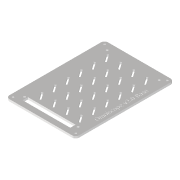
# Autodesk Inventor part: Omniscope_2.0_Base
Saved by Autodesk Inventor 2022 (Build 260153000, 153)
## iProperties
Created: 2022-05-25
Part Number: Omniscope_2.0_Base
Material: Generisch
Document SubType Name: Modeling
Designer: diederichbenedict
Density: 1 g/cm^3
Appearance: Vorgabe
Author: diederichbenedict
Autodesk Inventor part; units mm, degrees
ref_plane "YZ Plane" through (0, 0, 0) normal (1, 0, 0) x (0, 1, 0)
ref_plane "XZ Plane" through (0, 0, 0) normal (0, 1, 0) x (-1, 0, 0)
ref_plane "XY Plane" through (0, 0, 0) normal (0, 0, 1) x (1, 0, 0)
sketch "Skizze1" plane through (0, 0, 0) normal (0, 1, 0) x (-1, 0, 0)
  line L0 (-42.75, -63.75) -> (42.75, -63.75)
  line L1 (42.75, -63.75) -> (42.75, 63.75)
  line L2 (42.75, 63.75) -> (-42.75, 63.75)
  line L3 (-42.75, 63.75) -> (-42.75, -63.75)
  line L4 (-42.75, -63.75) -> (42.75, 63.75) construction
  line L5 (42.75, -63.75) -> (-42.75, 63.75) construction
  line L6 (46.7304, -64.3892) -> (-44.1, -64.3892) projected
  line L7 (46.7304, 68.4528) -> (46.7304, -64.3892) projected
  line L8 (-44.1, 68.4528) -> (46.7304, 68.4528) projected
  line L9 (-44.1, -64.3892) -> (-44.1, 68.4528) projected
  circle A0 centre (-37.9024, -58.852) radius 1.6 projected
  circle A1 centre (-37.75, 58.75) radius 1.6 projected
  circle A2 centre (-30.897, 60.7312) radius 0.5 construction
  circle A3 centre (-28.357, 60.7312) radius 0.5 construction
  circle A4 centre (-25.4992, 60.7312) radius 0.5 construction
  circle A5 centre (-22.9592, 60.7312) radius 0.5 construction
  circle A6 centre (-12.1431, 60.8071) radius 0.5 construction
  circle A7 centre (-9.6031, 60.8071) radius 0.5 construction
  circle A8 centre (-6.7453, 60.8071) radius 0.5 construction
  circle A9 centre (-4.2053, 60.8071) radius 0.5 construction
  circle A10 centre (28.29, -47.2696) radius 1.6 projected
  circle A11 centre (37.5356, -58.7504) radius 1.6 projected
  circle A12 centre (6.8561, 60.8071) radius 0.5 construction
  circle A13 centre (9.3961, 60.8071) radius 0.5 construction
  circle A14 centre (12.2539, 60.8071) radius 0.5 construction
  circle A15 centre (14.7939, 60.8071) radius 0.5 construction
  circle A16 centre (25.7537, 60.8579) radius 0.5 construction
  circle A17 centre (28.2937, 60.8579) radius 0.5 construction
  circle A18 centre (31.1515, 60.8579) radius 0.5 construction
  circle A19 centre (33.6915, 60.8579) radius 0.5 construction
  circle A20 centre (38.9072, 59.8168) radius 1.6 projected
  line L10 (46.7304, -69.3892) -> (-44.1, -69.3892)
  line L11 (-49.1, -64.3892) -> (-49.1, 68.4528)
  line L12 (-44.1, 73.4528) -> (46.7304, 73.4528)
  line L13 (51.7304, 68.4528) -> (51.7304, -64.3892)
  arc A21 (51.7304, 68.4528) -> (46.7304, 73.4528) centre (46.7304, 68.4528) ccw
  arc A22 (-44.1, 73.4528) -> (-49.1, 68.4528) centre (-44.1, 68.4528) ccw
  arc A23 (-49.1, -64.3892) -> (-44.1, -69.3892) centre (-44.1, -64.3892) ccw
  arc A24 (46.7304, -69.3892) -> (51.7304, -64.3892) centre (46.7304, -64.3892) ccw
  line L14 (-33.3052, 57.5577) -> (35.9356, 57.5577)
  line L15 (35.9356, 57.5577) -> (35.9356, 65.2759)
  line L16 (35.9356, 65.2759) -> (-33.3052, 65.2759)
  line L17 (-33.3052, 65.2759) -> (-33.3052, 57.5577)
  line L18 (-33.3052, 57.5577) -> (35.9356, 65.2759) construction
  line L19 (35.9356, 57.5577) -> (-33.3052, 65.2759) construction
  point P0 (0, 0)
  point P1 (1.3152, 61.4168)
  dimension "d0" = 85.5
  dimension "d1" = 127.5
  dimension "d47" = 5
  dimension "d48" = 5
  constraints: 32 end point, 8 point on circle, 8 tangent, 4 centre point, 4 midpoint, 4 parallel, 3 equal radius, 2 horizontal, 2 perpendicular, 3 other
  measures "d0" distance of L2.end L1.end
  measures "d1" distance of L1.end L0.end
  measures "d47" distance between parallel lines of L7 L13
  measures "d48" radius of A21
extrude "Extrusion1" add sketch "Skizze1" along normal blind 3 contours L3 L2 L17 L14 L15 L1 L0 | L6 L9 L8 L7 | A10 | L10 A23 L11 A22 L12 A21 L13 A24
sketch "Skizze8" plane through (0, 3, 0) normal (0, 1, 0) x (1, 0, 0)
  circle A0 centre (-28.29, 47.2696) radius 1.6 projected
  line L0 (-46.7304, -73.4528) -> (44.1, -73.4528) projected
  arc A1 (44.1, -73.4528) -> (49.1, -68.4528) centre (44.1, -68.4528) ccw projected
  line L1 (49.1, -68.4528) -> (49.1, 64.3892) projected
  arc A2 (49.1, 64.3892) -> (44.1, 69.3892) centre (44.1, 64.3892) ccw projected
  line L2 (44.1, 69.3892) -> (-46.7304, 69.3892) projected
  arc A3 (-46.7304, 69.3892) -> (-51.7304, 64.3892) centre (-46.7304, 64.3892) ccw projected
  line L3 (-51.7304, 64.3892) -> (-51.7304, -68.4528) projected
  arc A4 (-51.7304, -68.4528) -> (-46.7304, -73.4528) centre (-46.7304, -68.4528) ccw projected
  line L4 (-32.7356, 53.5165) -> (-24.8933, 42.3165)
  line L5 (-24.8933, 42.3165) -> (-22.8454, 43.7504)
  line L6 (-22.8454, 43.7504) -> (-30.6877, 54.9504)
  line L7 (-30.6877, 54.9504) -> (-32.7356, 53.5165)
  line L8 (-32.7356, 53.5165) -> (-22.8454, 43.7504) construction
  line L9 (-24.8933, 42.3165) -> (-30.6877, 54.9504) construction
  line L10 (-32.7356, 53.5165) -> (-19.0629, 53.5165) construction
  circle A5 centre (-37.5356, 58.7504) radius 1.6 projected
  point P0 (0, 0)
  point P1 (-27.7905, 48.6334)
  dimension "d49" = 55
  dimension "d50" = 2.5
  dimension "d51" = 35
  dimension "d55" = 3.8
  dimension "d57" = 15
  dimension "d58" = 4.8
  constraints: 14 end point, 2 midpoint, 2 parallel, 1 equal length, 1 horizontal, 1 perpendicular
  measures "d49" angle of L4 L10
  measures "d50" distance of L5.end L4.end
  measures "d51" angle of L4 L3
  measures "d55" vertical distance of A5.centre L6.end
  measures "d57" vertical distance of A5.centre L5.end
  measures "d58" horizontal distance of L4.start A5.centre
extrude "Extrusion5" cut sketch "Skizze8" against normal through all contours A0 L4 | A0 L4 L7 L6 L5 picked at (-28.4041, 47.7742)
pattern_linear "Rechteckige Anordnung3" count 6 spacing 19 along (0, 0, 1) count 4 spacing 19 along (1, 0, 0) of "Extrusion5"
sketch "Skizze9" plane through (0, 3, 0) normal (0, 1, 0) x (1, 0, 0)
  line L0 (32.1067, -52.6835) -> (24.2644, -41.4835) projected
  line L1 (24.2644, -41.4835) -> (26.3123, -40.0496) projected
  line L2 (26.3123, -40.0496) -> (34.1546, -51.2496) projected
  line L3 (34.1546, -51.2496) -> (32.1067, -52.6835) projected
  line L4 (32.1067, -33.6835) -> (24.2644, -22.4835) projected
  line L5 (24.2644, -22.4835) -> (26.3123, -21.0496) projected
  line L6 (26.3123, -21.0496) -> (34.1546, -32.2496) projected
  line L7 (34.1546, -32.2496) -> (32.1067, -33.6835) projected
  line L8 (32.1067, -14.6835) -> (24.2644, -3.4835) projected
  line L9 (24.2644, -3.4835) -> (26.3123, -2.0496) projected
  line L10 (26.3123, -2.0496) -> (34.1546, -13.2496) projected
  line L11 (34.1546, -13.2496) -> (32.1067, -14.6835) projected
  line L12 (32.1067, 4.3165) -> (24.2644, 15.5165) projected
  line L13 (24.2644, 15.5165) -> (26.3123, 16.9504) projected
  line L14 (26.3123, 16.9504) -> (34.1546, 5.7504) projected
  line L15 (34.1546, 5.7504) -> (32.1067, 4.3165) projected
  line L16 (32.1067, 23.3165) -> (24.2644, 34.5165) projected
  line L17 (24.2644, 34.5165) -> (26.3123, 35.9504) projected
  line L18 (26.3123, 35.9504) -> (34.1546, 24.7504) projected
  line L19 (34.1546, 24.7504) -> (32.1067, 23.3165) projected
  line L20 (32.1067, 42.3165) -> (24.2644, 53.5165) projected
  line L21 (24.2644, 53.5165) -> (26.3123, 54.9504) projected
  line L22 (26.3123, 54.9504) -> (34.1546, 43.7504) projected
  line L23 (34.1546, 43.7504) -> (32.1067, 42.3165) projected
  line L24 (13.1067, -52.6835) -> (5.2644, -41.4835) projected
  line L25 (5.2644, -41.4835) -> (7.3123, -40.0496) projected
  line L26 (7.3123, -40.0496) -> (15.1546, -51.2496) projected
  line L27 (15.1546, -51.2496) -> (13.1067, -52.6835) projected
  line L28 (13.1067, -33.6835) -> (5.2644, -22.4835) projected
  line L29 (5.2644, -22.4835) -> (7.3123, -21.0496) projected
  line L30 (7.3123, -21.0496) -> (15.1546, -32.2496) projected
  line L31 (15.1546, -32.2496) -> (13.1067, -33.6835) projected
  line L32 (13.1067, -14.6835) -> (5.2644, -3.4835) projected
  line L33 (5.2644, -3.4835) -> (7.3123, -2.0496) projected
  line L34 (7.3123, -2.0496) -> (15.1546, -13.2496) projected
  line L35 (15.1546, -13.2496) -> (13.1067, -14.6835) projected
  line L36 (13.1067, 4.3165) -> (5.2644, 15.5165) projected
  line L37 (5.2644, 15.5165) -> (7.3123, 16.9504) projected
  line L38 (7.3123, 16.9504) -> (15.1546, 5.7504) projected
  line L39 (15.1546, 5.7504) -> (13.1067, 4.3165) projected
  line L40 (13.1067, 23.3165) -> (5.2644, 34.5165) projected
  line L41 (5.2644, 34.5165) -> (7.3123, 35.9504) projected
  line L42 (7.3123, 35.9504) -> (15.1546, 24.7504) projected
  line L43 (15.1546, 24.7504) -> (13.1067, 23.3165) projected
  line L44 (13.1067, 42.3165) -> (5.2644, 53.5165) projected
  line L45 (5.2644, 53.5165) -> (7.3123, 54.9504) projected
  line L46 (7.3123, 54.9504) -> (15.1546, 43.7504) projected
  line L47 (15.1546, 43.7504) -> (13.1067, 42.3165) projected
  line L48 (-5.8933, -52.6835) -> (-13.7356, -41.4835) projected
  line L49 (-13.7356, -41.4835) -> (-11.6877, -40.0496) projected
  line L50 (-11.6877, -40.0496) -> (-3.8454, -51.2496) projected
  line L51 (-3.8454, -51.2496) -> (-5.8933, -52.6835) projected
  line L52 (-5.8933, -33.6835) -> (-13.7356, -22.4835) projected
  line L53 (-13.7356, -22.4835) -> (-11.6877, -21.0496) projected
  line L54 (-11.6877, -21.0496) -> (-3.8454, -32.2496) projected
  line L55 (-3.8454, -32.2496) -> (-5.8933, -33.6835) projected
  line L56 (-5.8933, -14.6835) -> (-13.7356, -3.4835) projected
  line L57 (-13.7356, -3.4835) -> (-11.6877, -2.0496) projected
  line L58 (-11.6877, -2.0496) -> (-3.8454, -13.2496) projected
  line L59 (-3.8454, -13.2496) -> (-5.8933, -14.6835) projected
  line L60 (-5.8933, 4.3165) -> (-13.7356, 15.5165) projected
  line L61 (-13.7356, 15.5165) -> (-11.6877, 16.9504) projected
  line L62 (-11.6877, 16.9504) -> (-3.8454, 5.7504) projected
  line L63 (-3.8454, 5.7504) -> (-5.8933, 4.3165) projected
  line L64 (-5.8933, 23.3165) -> (-13.7356, 34.5165) projected
  line L65 (-13.7356, 34.5165) -> (-11.6877, 35.9504) projected
  line L66 (-11.6877, 35.9504) -> (-3.8454, 24.7504) projected
  line L67 (-3.8454, 24.7504) -> (-5.8933, 23.3165) projected
  line L68 (-5.8933, 42.3165) -> (-13.7356, 53.5165) projected
  line L69 (-13.7356, 53.5165) -> (-11.6877, 54.9504) projected
  line L70 (-11.6877, 54.9504) -> (-3.8454, 43.7504) projected
  line L71 (-3.8454, 43.7504) -> (-5.8933, 42.3165) projected
  line L72 (-24.8933, -52.6835) -> (-32.7356, -41.4835) projected
  line L73 (-32.7356, -41.4835) -> (-30.6877, -40.0496) projected
  line L74 (-30.6877, -40.0496) -> (-22.8454, -51.2496) projected
  line L75 (-22.8454, -51.2496) -> (-24.8933, -52.6835) projected
  line L76 (-24.8933, -33.6835) -> (-32.7356, -22.4835) projected
  line L77 (-32.7356, -22.4835) -> (-30.6877, -21.0496) projected
  line L78 (-30.6877, -21.0496) -> (-22.8454, -32.2496) projected
  line L79 (-22.8454, -32.2496) -> (-24.8933, -33.6835) projected
  line L80 (-24.8933, -14.6835) -> (-32.7356, -3.4835) projected
  line L81 (-32.7356, -3.4835) -> (-30.6877, -2.0496) projected
  line L82 (-30.6877, -2.0496) -> (-22.8454, -13.2496) projected
  line L83 (-22.8454, -13.2496) -> (-24.8933, -14.6835) projected
  line L84 (-24.8933, 4.3165) -> (-32.7356, 15.5165) projected
  line L85 (-32.7356, 15.5165) -> (-30.6877, 16.9504) projected
  line L86 (-30.6877, 16.9504) -> (-22.8454, 5.7504) projected
  line L87 (-22.8454, 5.7504) -> (-24.8933, 4.3165) projected
  line L88 (-24.8933, 23.3165) -> (-32.7356, 34.5165) projected
  line L89 (-32.7356, 34.5165) -> (-30.6877, 35.9504) projected
  line L90 (-30.6877, 35.9504) -> (-22.8454, 24.7504) projected
  line L91 (-22.8454, 24.7504) -> (-24.8933, 23.3165) projected
  line L92 (-30.6877, 54.9504) -> (-22.8454, 43.7504) projected
  line L93 (-22.8454, 43.7504) -> (-24.8933, 42.3165) projected
  line L94 (-24.8933, 42.3165) -> (-32.7356, 53.5165) projected
  line L95 (-32.7356, 53.5165) -> (-30.6877, 54.9504) projected
  line L96 (-46.7304, -73.4528) -> (44.1, -73.4528) projected
  arc A0 (44.1, -73.4528) -> (49.1, -68.4528) centre (44.1, -68.4528) ccw projected
  line L97 (49.1, -68.4528) -> (49.1, 64.3892) projected
  arc A1 (49.1, 64.3892) -> (44.1, 69.3892) centre (44.1, 64.3892) ccw projected
  line L98 (44.1, 69.3892) -> (-46.7304, 69.3892) projected
  arc A2 (-46.7304, 69.3892) -> (-51.7304, 64.3892) centre (-46.7304, 64.3892) ccw projected
  line L99 (-51.7304, 64.3892) -> (-51.7304, -68.4528) projected
  arc A3 (-51.7304, -68.4528) -> (-46.7304, -73.4528) centre (-46.7304, -68.4528) ccw projected
  circle A4 centre (-38.9072, -59.8168) radius 1.6 projected
  circle A5 centre (-37.5356, 58.7504) radius 1.6 projected
  circle A6 centre (37.75, -58.75) radius 1.6 projected
  circle A7 centre (37.9024, 58.852) radius 1.6 projected
  line L100 (33.3052, -57.5577) -> (33.3052, -65.2759) projected
  line L101 (33.3052, -65.2759) -> (-35.9356, -65.2759) projected
  line L102 (-35.9356, -65.2759) -> (-35.9356, -57.5577) projected
  line L103 (-35.9356, -57.5577) -> (33.3052, -57.5577) projected
  point P0 (0, 0)
hole "Bohrung3" at (44.1, 3, 68.4528) at (44.1, 3, -64.3892) at (-46.7304, 3, -64.3892) at (-46.7304, 3, 68.4528) direction (0, -1, 0) diameter 2.8 depth 14 tip angle 118
sketch "Skizze10" plane through (0, 3, 0) normal (0, 1, 0) x (1, 0, 0)
  line L0 (38.6334, -37.4624) -> (38.6334, 40.4783) construction
  line L1 (38.6334, 40.4783) -> (46.1532, 40.4783) construction
  line L2 (46.1532, 40.4783) -> (46.1532, -37.4624) construction
  line L3 (46.1532, -37.4624) -> (38.6334, -37.4624) construction
  spline S0 degree 2 poles (39.4178, -32.7749) (39.8029, -32.4461) (40.9302, -32.0798) (41.6535, -32.0798) knots 0 0 0 1 2 2 2
  spline S1 degree 2 poles (41.6535, -32.0798) (42.3581, -32.0798) (43.4994, -32.4367) (43.8846, -32.7749) knots 0 0 0 1 2 2 2
  spline S2 degree 2 poles (43.8846, -32.7749) (44.2885, -33.1319) (44.6736, -34.0759) (44.6736, -34.6443) knots 0 0 0 1 2 2 2
  spline S3 degree 2 poles (44.6736, -34.6443) (44.6736, -35.2314) (44.2744, -36.1708) (43.8846, -36.5136) knots 0 0 0 1 2 2 2
  spline S4 degree 2 poles (43.8846, -36.5136) (43.4994, -36.8471) (42.3674, -37.2041) (41.6535, -37.2041) knots 0 0 0 1 2 2 2
  spline S5 degree 2 poles (41.6535, -37.2041) (40.9255, -37.2041) (39.817, -36.8424) (39.4178, -36.5089) knots 0 0 0 1 2 2 2
  spline S6 degree 2 poles (39.4178, -36.5089) (39.0326, -36.1708) (38.6334, -35.2267) (38.6334, -34.6443) knots 0 0 0 1 2 2 2
  spline S7 degree 2 poles (38.6334, -34.6443) (38.6334, -34.0525) (39.0467, -33.1037) (39.4178, -32.7749) knots 0 0 0 1 2 2 2
  spline S8 degree 2 poles (41.6535, -32.8829) (41.0805, -32.8829) (40.1928, -33.1319) (39.9016, -33.3573) knots 0 0 0 1 2 2 2
  spline S9 degree 2 poles (39.9016, -33.3573) (39.601, -33.5875) (39.3004, -34.2356) (39.3004, -34.6396) knots 0 0 0 1 2 2 2
  spline S10 degree 2 poles (39.3004, -34.6396) (39.3004, -35.0576) (39.5916, -35.687) (39.9016, -35.9265) knots 0 0 0 1 2 2 2
  spline S11 degree 2 poles (39.9016, -35.9265) (40.1975, -36.1567) (41.0899, -36.4009) (41.6535, -36.4009) knots 0 0 0 1 2 2 2
  spline S12 degree 2 poles (41.6535, -36.4009) (42.7949, -36.4009) (44.0067, -35.4427) (44.0067, -34.6396) knots 0 0 0 1 2 2 2
  spline S13 degree 2 poles (44.0067, -34.6396) (44.0067, -33.8364) (42.7949, -32.8829) (41.6535, -32.8829) knots 0 0 0 1 2 2 2
  line L4 (44.5515, -26.3589) -> (42.034, -26.3589)
  spline S14 degree 2 poles (42.034, -26.3589) (41.7334, -26.3589) (41.2214, -26.4059) (41.0805, -26.481) knots 0 0 0 1 2 2 2
  spline S15 degree 2 poles (41.0805, -26.481) (40.9255, -26.5562) (40.7752, -26.8427) (40.7752, -27.0916) knots 0 0 0 1 2 2 2
  spline S16 degree 2 poles (40.7752, -27.0916) (40.7752, -27.3171) (41.0523, -27.8337) (41.3153, -28.1062) knots 0 0 0 1 2 2 2
  spline S17 degree 2 poles (41.3153, -28.1062) (41.3811, -28.1015) (41.5643, -28.0921) (41.6864, -28.0921) knots 0 0 0 1 2 2 2
  line L5 (41.6864, -28.0921) -> (44.5515, -28.0921)
  line L6 (44.5515, -28.0921) -> (44.5515, -28.8248)
  line L7 (44.5515, -28.8248) -> (42.034, -28.8248)
  spline S18 degree 2 poles (42.034, -28.8248) (41.7334, -28.8248) (41.2214, -28.8718) (41.0805, -28.9469) knots 0 0 0 1 2 2 2
  spline S19 degree 2 poles (41.0805, -28.9469) (40.9255, -29.0221) (40.7752, -29.3086) (40.7752, -29.5575) knots 0 0 0 1 2 2 2
  spline S20 degree 2 poles (40.7752, -29.5575) (40.7752, -29.7924) (41.0711, -30.3137) (41.3012, -30.558) knots 0 0 0 1 2 2 2
  line L8 (41.3012, -30.558) -> (44.5515, -30.558)
  line L9 (44.5515, -30.558) -> (44.5515, -31.2907)
  line L10 (44.5515, -31.2907) -> (40.2022, -31.2907)
  line L11 (40.2022, -31.2907) -> (40.2022, -30.558)
  line L12 (40.2022, -30.558) -> (40.6813, -30.558)
  spline S21 degree 2 poles (40.6813, -30.558) (40.3947, -30.2714) (40.08, -29.7078) (40.08, -29.3696) knots 0 0 0 1 2 2 2
  spline S22 degree 2 poles (40.08, -29.3696) (40.08, -28.9845) (40.4323, -28.388) (40.8316, -28.233) knots 0 0 0 1 2 2 2
  spline S23 degree 2 poles (40.8316, -28.233) (40.4605, -27.8995) (40.08, -27.2701) (40.08, -26.9037) knots 0 0 0 1 2 2 2
  spline S24 degree 2 poles (40.08, -26.9037) (40.08, -26.6219) (40.2538, -26.1616) (40.4511, -25.9925) knots 0 0 0 1 2 2 2
  spline S25 degree 2 poles (40.4511, -25.9925) (40.6484, -25.8188) (41.2402, -25.6262) (41.6864, -25.6262) knots 0 0 0 1 2 2 2
  line L13 (41.6864, -25.6262) -> (44.5515, -25.6262)
  line L14 (44.5515, -25.6262) -> (44.5515, -26.3589)
  line L15 (44.5515, -21.1829) -> (44.5515, -21.9156)
  line L16 (44.5515, -21.9156) -> (42.0715, -21.9156)
  spline S26 degree 2 poles (42.0715, -21.9156) (41.7709, -21.9156) (41.2543, -21.972) (41.0993, -22.0565) knots 0 0 0 1 2 2 2
  spline S27 degree 2 poles (41.0993, -22.0565) (40.9349, -22.1458) (40.7752, -22.4652) (40.7752, -22.7376) knots 0 0 0 1 2 2 2
  spline S28 degree 2 poles (40.7752, -22.7376) (40.7752, -23.01) (41.0664, -23.5877) (41.3012, -23.8648) knots 0 0 0 1 2 2 2
  line L17 (41.3012, -23.8648) -> (44.5515, -23.8648)
  line L18 (44.5515, -23.8648) -> (44.5515, -24.5976)
  line L19 (44.5515, -24.5976) -> (40.2022, -24.5976)
  line L20 (40.2022, -24.5976) -> (40.2022, -23.8648)
  line L21 (40.2022, -23.8648) -> (40.686, -23.8648)
  spline S29 degree 2 poles (40.686, -23.8648) (40.39, -23.5361) (40.08, -22.902) (40.08, -22.545) knots 0 0 0 1 2 2 2
  spline S30 degree 2 poles (40.08, -22.545) (40.08, -21.9062) (40.9255, -21.1829) (41.7287, -21.1829) knots 0 0 0 1 2 2 2
  line L22 (41.7287, -21.1829) -> (44.5515, -21.1829)
  line L23 (44.5515, -19.4075) -> (44.5515, -20.1402)
  line L24 (44.5515, -20.1402) -> (40.2022, -20.1402)
  line L25 (40.2022, -20.1402) -> (40.2022, -19.4075)
  line L26 (40.2022, -19.4075) -> (44.5515, -19.4075)
  line L27 (39.4788, -19.3558) -> (39.4788, -20.1872)
  line L28 (39.4788, -20.1872) -> (38.7179, -20.1872)
  line L29 (38.7179, -20.1872) -> (38.7179, -19.3558)
  line L30 (38.7179, -19.3558) -> (39.4788, -19.3558)
  spline S31 degree 2 poles (44.6548, -17.1576) (44.6548, -17.5945) (44.42, -18.3507) (44.2885, -18.5996) knots 0 0 0 1 2 2 2
  line L31 (44.2885, -18.5996) -> (43.4665, -18.5996)
  line L32 (43.4665, -18.5996) -> (43.4665, -18.562)
  spline S32 degree 2 poles (43.4665, -18.562) (43.5417, -18.4681) (43.7202, -18.2144) (43.8188, -18.0031) knots 0 0 0 1 2 2 2
  spline S33 degree 2 poles (43.8188, -18.0031) (43.908, -17.8199) (44.0396, -17.369) (44.0396, -17.1295) knots 0 0 0 1 2 2 2
  spline S34 degree 2 poles (44.0396, -17.1295) (44.0396, -16.9557) (43.9597, -16.5564) (43.8939, -16.4625) knots 0 0 0 1 2 2 2
  spline S35 degree 2 poles (43.8939, -16.4625) (43.8047, -16.3263) (43.6027, -16.2042) (43.3961, -16.2042) knots 0 0 0 1 2 2 2
  spline S36 degree 2 poles (43.3961, -16.2042) (43.1377, -16.2042) (42.87, -16.486) (42.7808, -16.8476) knots 0 0 0 1 2 2 2
  spline S37 degree 2 poles (42.7808, -16.8476) (42.7479, -16.9885) (42.654, -17.4395) (42.6023, -17.632) knots 0 0 0 1 2 2 2
  spline S38 degree 2 poles (42.6023, -17.632) (42.4567, -18.1299) (41.8555, -18.5808) (41.4281, -18.5808) knots 0 0 0 1 2 2 2
  spline S39 degree 2 poles (41.4281, -18.5808) (40.8363, -18.5808) (40.0988, -17.6931) (40.0988, -16.9604) knots 0 0 0 1 2 2 2
  spline S40 degree 2 poles (40.0988, -16.9604) (40.0988, -16.5987) (40.2773, -15.866) (40.4135, -15.617) knots 0 0 0 1 2 2 2
  line L33 (40.4135, -15.617) -> (41.1979, -15.617)
  line L34 (41.1979, -15.617) -> (41.1979, -15.6546)
  spline S41 degree 2 poles (41.1979, -15.6546) (40.9725, -15.9364) (40.7141, -16.6222) (40.7141, -16.9745) knots 0 0 0 1 2 2 2
  spline S42 degree 2 poles (40.7141, -16.9745) (40.7141, -17.3361) (41.0194, -17.834) (41.3247, -17.834) knots 0 0 0 1 2 2 2
  spline S43 degree 2 poles (41.3247, -17.834) (41.6019, -17.834) (41.8696, -17.5381) (41.9541, -17.2093) knots 0 0 0 1 2 2 2
  spline S44 degree 2 poles (41.9541, -17.2093) (41.9964, -17.0496) (42.0809, -16.6457) (42.1326, -16.4249) knots 0 0 0 1 2 2 2
  spline S45 degree 2 poles (42.1326, -16.4249) (42.2547, -15.9458) (42.8137, -15.4574) (43.2974, -15.4574) knots 0 0 0 1 2 2 2
  spline S46 degree 2 poles (43.2974, -15.4574) (43.5793, -15.4574) (44.0771, -15.6781) (44.2603, -15.8942) knots 0 0 0 1 2 2 2
  spline S47 degree 2 poles (44.2603, -15.8942) (44.4529, -16.1243) (44.6548, -16.7114) (44.6548, -17.1576) knots 0 0 0 1 2 2 2
  spline S48 degree 2 poles (44.6502, -13.0478) (44.6502, -13.4987) (44.373, -14.2455) (44.0912, -14.5133) knots 0 0 0 1 2 2 2
  spline S49 degree 2 poles (44.0912, -14.5133) (43.8141, -14.781) (42.9593, -15.0769) (42.3862, -15.0769) knots 0 0 0 1 2 2 2
  spline S50 degree 2 poles (42.3862, -15.0769) (41.8132, -15.0769) (40.9772, -14.7716) (40.6953, -14.5133) knots 0 0 0 1 2 2 2
  spline S51 degree 2 poles (40.6953, -14.5133) (40.4088, -14.2549) (40.1035, -13.4893) (40.1035, -13.0478) knots 0 0 0 1 2 2 2
  spline S52 degree 2 poles (40.1035, -13.0478) (40.1035, -12.6909) (40.3055, -12.0239) (40.437, -11.7656) knots 0 0 0 1 2 2 2
  line L35 (40.437, -11.7656) -> (41.259, -11.7656)
  line L36 (41.259, -11.7656) -> (41.259, -11.8078)
  spline S53 degree 2 poles (41.259, -11.8078) (41.1932, -11.8877) (41.0241, -12.1319) (40.9349, -12.3057) knots 0 0 0 1 2 2 2
  spline S54 degree 2 poles (40.9349, -12.3057) (40.8597, -12.4607) (40.7423, -12.874) (40.7423, -13.0619) knots 0 0 0 1 2 2 2
  spline S55 degree 2 poles (40.7423, -13.0619) (40.7423, -13.6302) (41.6019, -14.3207) (42.3862, -14.3207) knots 0 0 0 1 2 2 2
  spline S56 degree 2 poles (42.3862, -14.3207) (43.1518, -14.3207) (44.0114, -13.6537) (44.0114, -13.0619) knots 0 0 0 1 2 2 2
  spline S57 degree 2 poles (44.0114, -13.0619) (44.0114, -12.705) (43.7155, -12.0568) (43.4853, -11.8078) knots 0 0 0 1 2 2 2
  line L37 (43.4853, -11.8078) -> (43.4853, -11.7656)
  line L38 (43.4853, -11.7656) -> (44.3073, -11.7656)
  spline S58 degree 2 poles (44.3073, -11.7656) (44.3589, -11.8736) (44.5045, -12.2024) (44.5374, -12.3339) knots 0 0 0 1 2 2 2
  spline S59 degree 2 poles (44.5374, -12.3339) (44.5938, -12.5218) (44.6502, -12.8177) (44.6502, -13.0478) knots 0 0 0 1 2 2 2
  spline S60 degree 2 poles (42.3768, -7.5243) (43.4759, -7.5243) (44.6736, -8.5811) (44.6736, -9.4641) knots 0 0 0 1 2 2 2
  spline S61 degree 2 poles (44.6736, -9.4641) (44.6736, -10.3706) (43.4383, -11.4086) (42.3768, -11.4086) knots 0 0 0 1 2 2 2
  spline S62 degree 2 poles (42.3768, -11.4086) (41.2872, -11.4086) (40.08, -10.3377) (40.08, -9.4641) knots 0 0 0 1 2 2 2
  spline S63 degree 2 poles (40.08, -9.4641) (40.08, -8.5811) (41.2825, -7.5243) (42.3768, -7.5243) knots 0 0 0 1 2 2 2
  spline S64 degree 2 poles (42.3768, -8.2805) (41.5314, -8.2805) (40.7094, -8.8958) (40.7094, -9.4641) knots 0 0 0 1 2 2 2
  spline S65 degree 2 poles (40.7094, -9.4641) (40.7094, -10.0324) (41.5314, -10.6524) (42.3768, -10.6524) knots 0 0 0 1 2 2 2
  spline S66 degree 2 poles (42.3768, -10.6524) (43.1988, -10.6524) (44.0442, -10.0324) (44.0442, -9.4641) knots 0 0 0 1 2 2 2
  spline S67 degree 2 poles (44.0442, -9.4641) (44.0442, -8.9005) (43.2129, -8.2805) (42.3768, -8.2805) knots 0 0 0 1 2 2 2
  spline S68 degree 2 poles (42.2594, -3.1279) (43.3491, -3.1279) (44.6361, -4.166) (44.6361, -4.9597) knots 0 0 0 1 2 2 2
  spline S69 degree 2 poles (44.6361, -4.9597) (44.6361, -5.2838) (44.4858, -5.7817) (44.3308, -6.04) knots 0 0 0 1 2 2 2
  line L39 (44.3308, -6.04) -> (46.1532, -6.04)
  line L40 (46.1532, -6.04) -> (46.1532, -6.7727)
  line L41 (46.1532, -6.7727) -> (40.2022, -6.7727)
  line L42 (40.2022, -6.7727) -> (40.2022, -6.04)
  line L43 (40.2022, -6.04) -> (40.6578, -6.04)
  spline S70 degree 2 poles (40.6578, -6.04) (40.4088, -5.7676) (40.08, -5.1006) (40.08, -4.7108) knots 0 0 0 1 2 2 2
  spline S71 degree 2 poles (40.08, -4.7108) (40.08, -3.964) (41.2637, -3.1279) (42.2594, -3.1279) knots 0 0 0 1 2 2 2
  spline S72 degree 2 poles (42.344, -3.8841) (41.5972, -3.8841) (40.7752, -4.3585) (40.7752, -4.8893) knots 0 0 0 1 2 2 2
  spline S73 degree 2 poles (40.7752, -4.8893) (40.7752, -5.1993) (41.0523, -5.7817) (41.2684, -6.04) knots 0 0 0 1 2 2 2
  line L44 (41.2684, -6.04) -> (43.7389, -6.04)
  spline S74 degree 2 poles (43.7389, -6.04) (43.8752, -5.7535) (43.9785, -5.3449) (43.9785, -5.0819) knots 0 0 0 1 2 2 2
  spline S75 degree 2 poles (43.9785, -5.0819) (43.9785, -4.5135) (43.1424, -3.8841) (42.344, -3.8841) knots 0 0 0 1 2 2 2
  spline S76 degree 2 poles (44.6502, -0.4789) (44.6502, -1.5216) (43.4806, -2.6676) (42.4003, -2.6676) knots 0 0 0 1 2 2 2
  spline S77 degree 2 poles (42.4003, -2.6676) (41.3388, -2.6676) (40.08, -1.5545) (40.08, -0.6574) knots 0 0 0 1 2 2 2
  spline S78 degree 2 poles (40.08, -0.6574) (40.08, -0.2534) (40.3149, 0.3713) (40.5638, 0.6014) knots 0 0 0 1 2 2 2
  spline S79 degree 2 poles (40.5638, 0.6014) (40.8128, 0.8363) (41.5314, 1.0852) (42.0528, 1.0852) knots 0 0 0 1 2 2 2
  line L45 (42.0528, 1.0852) -> (42.452, 1.0852)
  line L46 (42.452, 1.0852) -> (42.452, -1.9255)
  spline S80 degree 2 poles (42.452, -1.9255) (43.2082, -1.9255) (44.0114, -1.1646) (44.0114, -0.4883) knots 0 0 0 1 2 2 2
  spline S81 degree 2 poles (44.0114, -0.4883) (44.0114, -0.2487) (43.9033, 0.2163) (43.8188, 0.4041) knots 0 0 0 1 2 2 2
  spline S82 degree 2 poles (43.8188, 0.4041) (43.7249, 0.6014) (43.5605, 0.8738) (43.4853, 0.9631) knots 0 0 0 1 2 2 2
  line L47 (43.4853, 0.9631) -> (43.4853, 1.0054)
  line L48 (43.4853, 1.0054) -> (44.2838, 1.0054)
  spline S83 degree 2 poles (44.2838, 1.0054) (44.3355, 0.8785) (44.4858, 0.4934) (44.528, 0.3431) knots 0 0 0 1 2 2 2
  spline S84 degree 2 poles (44.528, 0.3431) (44.5891, 0.1317) (44.6502, -0.2158) (44.6502, -0.4789) knots 0 0 0 1 2 2 2
  spline S85 degree 2 poles (41.8931, 0.3713) (41.5972, 0.3619) (41.165, 0.2398) (41.0194, 0.1223) knots 0 0 0 1 2 2 2
  spline S86 degree 2 poles (41.0194, 0.1223) (40.855, -0.0045) (40.6813, -0.4037) (40.6813, -0.6996) knots 0 0 0 1 2 2 2
  spline S87 degree 2 poles (40.6813, -0.6996) (40.6813, -0.9908) (40.855, -1.3995) (41.0241, -1.5686) knots 0 0 0 1 2 2 2
  spline S88 degree 2 poles (41.0241, -1.5686) (41.1979, -1.7329) (41.6159, -1.902) (41.8931, -1.9255) knots 0 0 0 1 2 2 2
  line L49 (41.8931, -1.9255) -> (41.8931, 0.3713)
  line L50 (40.2022, 7.7313) -> (44.5515, 6.0921)
  line L51 (44.5515, 6.0921) -> (44.5515, 5.4346)
  line L52 (44.5515, 5.4346) -> (40.2022, 3.8094)
  line L53 (40.2022, 3.8094) -> (40.2022, 4.6032)
  line L54 (40.2022, 4.6032) -> (43.5511, 5.7915)
  line L55 (43.5511, 5.7915) -> (40.2022, 6.9704)
  line L56 (40.2022, 6.9704) -> (40.2022, 7.7313)
  line L57 (44.5515, 11.7519) -> (44.5515, 8.1776)
  line L58 (44.5515, 8.1776) -> (43.7296, 8.1776)
  spline S89 degree 2 poles (43.7296, 8.1776) (43.3679, 8.5627) (42.6962, 9.2484) (42.3346, 9.5772) knots 0 0 0 1 2 2 2
  spline S90 degree 2 poles (42.3346, 9.5772) (41.6065, 10.2395) (40.7329, 10.7233) (40.2679, 10.7233) knots 0 0 0 1 2 2 2
  spline S91 degree 2 poles (40.2679, 10.7233) (40.0237, 10.7233) (39.6573, 10.573) (39.5399, 10.4368) knots 0 0 0 1 2 2 2
  spline S92 degree 2 poles (39.5399, 10.4368) (39.4225, 10.3006) (39.3051, 9.9436) (39.3051, 9.7275) knots 0 0 0 1 2 2 2
  spline S93 degree 2 poles (39.3051, 9.7275) (39.3051, 9.5209) (39.4084, 9.0981) (39.4882, 8.9056) knots 0 0 0 1 2 2 2
  spline S94 degree 2 poles (39.4882, 8.9056) (39.554, 8.7412) (39.7419, 8.4359) (39.8076, 8.3419) knots 0 0 0 1 2 2 2
  line L59 (39.8076, 8.3419) -> (39.8076, 8.2997)
  line L60 (39.8076, 8.2997) -> (38.981, 8.2997)
  spline S95 degree 2 poles (38.981, 8.2997) (38.8635, 8.5392) (38.6334, 9.3988) (38.6334, 9.7839) knots 0 0 0 1 2 2 2
  spline S96 degree 2 poles (38.6334, 9.7839) (38.6334, 10.5965) (39.4929, 11.5124) (40.2257, 11.5124) knots 0 0 0 1 2 2 2
  spline S97 degree 2 poles (40.2257, 11.5124) (40.5685, 11.5124) (41.1416, 11.3527) (41.3858, 11.2118) knots 0 0 0 1 2 2 2
  spline S98 degree 2 poles (41.3858, 11.2118) (41.6394, 11.0709) (42.1373, 10.6622) (42.3768, 10.4368) knots 0 0 0 1 2 2 2
  spline S99 degree 2 poles (42.3768, 10.4368) (42.7761, 10.0704) (43.6309, 9.1733) (43.8799, 8.9056) knots 0 0 0 1 2 2 2
  line L61 (43.8799, 8.9056) -> (43.8799, 11.7519)
  line L62 (43.8799, 11.7519) -> (44.5515, 11.7519)
  line L63 (44.5515, 13.7716) -> (44.5515, 12.8416)
  line L64 (44.5515, 12.8416) -> (43.443, 12.8416)
  line L65 (43.443, 12.8416) -> (43.443, 13.7716)
  line L66 (43.443, 13.7716) -> (44.5515, 13.7716)
  spline S100 degree 2 poles (41.6535, 18.5484) (43.2129, 18.5484) (44.6736, 17.6418) (44.6736, 16.6978) knots 0 0 0 1 2 2 2
  spline S101 degree 2 poles (44.6736, 16.6978) (44.6736, 15.7396) (43.1847, 14.8425) (41.6582, 14.8425) knots 0 0 0 1 2 2 2
  spline S102 degree 2 poles (41.6582, 14.8425) (40.0894, 14.8425) (38.6381, 15.749) (38.6381, 16.6978) knots 0 0 0 1 2 2 2
  spline S103 degree 2 poles (38.6381, 16.6978) (38.6381, 17.6512) (40.1411, 18.5484) (41.6535, 18.5484) knots 0 0 0 1 2 2 2
  spline S104 degree 2 poles (43.4196, 17.5526) (43.133, 17.6653) (42.25, 17.7593) (41.6535, 17.7593) knots 0 0 0 1 2 2 2
  spline S105 degree 2 poles (41.6535, 17.7593) (41.057, 17.7593) (40.1787, 17.6653) (39.8828, 17.5479) knots 0 0 0 1 2 2 2
  spline S106 degree 2 poles (39.8828, 17.5479) (39.5869, 17.4305) (39.2816, 17.0219) (39.2816, 16.6978) knots 0 0 0 1 2 2 2
  spline S107 degree 2 poles (39.2816, 16.6978) (39.2816, 16.3737) (39.5869, 15.9557) (39.8922, 15.8335) knots 0 0 0 1 2 2 2
  spline S108 degree 2 poles (39.8922, 15.8335) (40.1881, 15.7161) (41.0899, 15.6316) (41.6582, 15.6316) knots 0 0 0 1 2 2 2
  spline S109 degree 2 poles (41.6582, 15.6316) (42.2688, 15.6316) (43.0861, 15.7067) (43.4055, 15.8288) knots 0 0 0 1 2 2 2
  spline S110 degree 2 poles (43.4055, 15.8288) (43.7061, 15.9416) (44.0302, 16.3596) (44.0302, 16.6978) knots 0 0 0 1 2 2 2
  spline S111 degree 2 poles (44.0302, 16.6978) (44.0302, 17.0172) (43.7249, 17.4352) (43.4196, 17.5526) knots 0 0 0 1 2 2 2
  spline S112 degree 2 poles (42.7714, 25.8755) (43.2035, 25.8755) (43.8658, 25.5468) (44.0818, 25.2743) knots 0 0 0 1 2 2 2
  spline S113 degree 2 poles (44.0818, 25.2743) (44.3355, 24.9456) (44.5515, 24.1987) (44.5515, 23.6069) knots 0 0 0 1 2 2 2
  line L67 (44.5515, 23.6069) -> (44.5515, 21.9442)
  line L68 (44.5515, 21.9442) -> (38.7555, 21.9442)
  line L69 (38.7555, 21.9442) -> (38.7555, 23.4801)
  spline S114 degree 2 poles (38.7555, 23.4801) (38.7555, 24.1001) (38.8354, 24.7201) (38.9904, 25.0019) knots 0 0 0 1 2 2 2
  spline S115 degree 2 poles (38.9904, 25.0019) (39.1548, 25.3166) (39.6949, 25.6031) (40.0613, 25.6031) knots 0 0 0 1 2 2 2
  spline S116 degree 2 poles (40.0613, 25.6031) (40.4699, 25.6031) (41.1181, 25.171) (41.3012, 24.7906) knots 0 0 0 1 2 2 2
  line L70 (41.3012, 24.7906) -> (41.3294, 24.7906)
  spline S117 degree 2 poles (41.3294, 24.7906) (41.4703, 25.3072) (42.2171, 25.8755) (42.7714, 25.8755) knots 0 0 0 1 2 2 2
  spline S118 degree 2 poles (42.8043, 25.0724) (42.4755, 25.0724) (42.0528, 24.8845) (41.9025, 24.6027) knots 0 0 0 1 2 2 2
  spline S119 degree 2 poles (41.9025, 24.6027) (41.8085, 24.4195) (41.7522, 23.9874) (41.7522, 23.5881) knots 0 0 0 1 2 2 2
  line L71 (41.7522, 23.5881) -> (41.7522, 22.7145)
  line L72 (41.7522, 22.7145) -> (43.8939, 22.7145)
  line L73 (43.8939, 22.7145) -> (43.8939, 23.3392)
  spline S120 degree 2 poles (43.8939, 23.3392) (43.8939, 23.8465) (43.8, 24.4289) (43.6497, 24.6543) knots 0 0 0 1 2 2 2
  spline S121 degree 2 poles (43.6497, 24.6543) (43.4947, 24.8704) (43.1096, 25.0724) (42.8043, 25.0724) knots 0 0 0 1 2 2 2
  spline S122 degree 2 poles (40.1693, 24.8) (39.9626, 24.8) (39.6526, 24.659) (39.5634, 24.504) knots 0 0 0 1 2 2 2
  spline S123 degree 2 poles (39.5634, 24.504) (39.4601, 24.3162) (39.4131, 23.8606) (39.4131, 23.4519) knots 0 0 0 1 2 2 2
  line L74 (39.4131, 23.4519) -> (39.4131, 22.7145)
  line L75 (39.4131, 22.7145) -> (41.1087, 22.7145)
  line L76 (41.1087, 22.7145) -> (41.1087, 23.5881)
  spline S124 degree 2 poles (41.1087, 23.5881) (41.1087, 23.9498) (41.0335, 24.2927) (40.9161, 24.4759) knots 0 0 0 1 2 2 2
  spline S125 degree 2 poles (40.9161, 24.4759) (40.8034, 24.6543) (40.4417, 24.8) (40.1693, 24.8) knots 0 0 0 1 2 2 2
  spline S126 degree 2 poles (44.0912, 29.0084) (44.157, 28.9192) (44.3918, 28.6185) (44.4623, 28.4776) knots 0 0 0 1 2 2 2
  spline S127 degree 2 poles (44.4623, 28.4776) (44.5656, 28.2851) (44.6736, 27.9234) (44.6736, 27.5946) knots 0 0 0 1 2 2 2
  spline S128 degree 2 poles (44.6736, 27.5946) (44.6736, 27.3269) (44.4717, 26.8431) (44.2885, 26.6599) knots 0 0 0 1 2 2 2
  spline S129 degree 2 poles (44.2885, 26.6599) (44.11, 26.4861) (43.584, 26.2748) (43.2927, 26.2748) knots 0 0 0 1 2 2 2
  spline S130 degree 2 poles (43.2927, 26.2748) (42.8418, 26.2748) (42.2031, 26.6552) (42.0199, 27.0686) knots 0 0 0 1 2 2 2
  spline S131 degree 2 poles (42.0199, 27.0686) (41.8508, 27.4349) (41.724, 28.4307) (41.6911, 29.0084) knots 0 0 0 1 2 2 2
  line L77 (41.6911, 29.0084) -> (41.5502, 29.0084)
  spline S132 degree 2 poles (41.5502, 29.0084) (41.2966, 29.0084) (40.9819, 28.8534) (40.8926, 28.7125) knots 0 0 0 1 2 2 2
  spline S133 degree 2 poles (40.8926, 28.7125) (40.8034, 28.5716) (40.747, 28.1676) (40.747, 27.9516) knots 0 0 0 1 2 2 2
  spline S134 degree 2 poles (40.747, 27.9516) (40.747, 27.698) (40.8973, 27.0122) (41.0429, 26.6693) knots 0 0 0 1 2 2 2
  line L78 (41.0429, 26.6693) -> (41.0429, 26.6271)
  line L79 (41.0429, 26.6271) -> (40.2961, 26.6271)
  spline S135 degree 2 poles (40.2961, 26.6271) (40.2397, 26.829) (40.0988, 27.5852) (40.0988, 27.9563) knots 0 0 0 1 2 2 2
  spline S136 degree 2 poles (40.0988, 27.9563) (40.0988, 28.4072) (40.2397, 29.0225) (40.4229, 29.2667) knots 0 0 0 1 2 2 2
  spline S137 degree 2 poles (40.4229, 29.2667) (40.6014, 29.5063) (41.1697, 29.7411) (41.5784, 29.7411) knots 0 0 0 1 2 2 2
  line L80 (41.5784, 29.7411) -> (44.5515, 29.7411)
  line L81 (44.5515, 29.7411) -> (44.5515, 29.0084)
  line L82 (44.5515, 29.0084) -> (44.0912, 29.0084)
  line L83 (43.4806, 29.0084) -> (42.2735, 29.0084)
  spline S138 degree 2 poles (42.2735, 29.0084) (42.297, 28.7454) (42.3768, 27.9516) (42.452, 27.7027) knots 0 0 0 1 2 2 2
  spline S139 degree 2 poles (42.452, 27.7027) (42.5412, 27.4114) (42.9123, 27.031) (43.2411, 27.031) knots 0 0 0 1 2 2 2
  spline S140 degree 2 poles (43.2411, 27.031) (43.6168, 27.031) (43.9973, 27.4537) (43.9973, 27.8576) knots 0 0 0 1 2 2 2
  spline S141 degree 2 poles (43.9973, 27.8576) (43.9973, 28.2005) (43.7014, 28.7642) (43.4806, 29.0084) knots 0 0 0 1 2 2 2
  spline S142 degree 2 poles (44.6548, 31.944) (44.6548, 31.5072) (44.42, 30.751) (44.2885, 30.502) knots 0 0 0 1 2 2 2
  line L84 (44.2885, 30.502) -> (43.4665, 30.502)
  line L85 (43.4665, 30.502) -> (43.4665, 30.5396)
  spline S143 degree 2 poles (43.4665, 30.5396) (43.5417, 30.6335) (43.7202, 30.8872) (43.8188, 31.0985) knots 0 0 0 1 2 2 2
  spline S144 degree 2 poles (43.8188, 31.0985) (43.908, 31.2817) (44.0396, 31.7326) (44.0396, 31.9722) knots 0 0 0 1 2 2 2
  spline S145 degree 2 poles (44.0396, 31.9722) (44.0396, 32.1459) (43.9597, 32.5452) (43.8939, 32.6391) knots 0 0 0 1 2 2 2
  spline S146 degree 2 poles (43.8939, 32.6391) (43.8047, 32.7753) (43.6027, 32.8974) (43.3961, 32.8974) knots 0 0 0 1 2 2 2
  spline S147 degree 2 poles (43.3961, 32.8974) (43.1377, 32.8974) (42.87, 32.6156) (42.7808, 32.254) knots 0 0 0 1 2 2 2
  spline S148 degree 2 poles (42.7808, 32.254) (42.7479, 32.1131) (42.654, 31.6622) (42.6023, 31.4696) knots 0 0 0 1 2 2 2
  spline S149 degree 2 poles (42.6023, 31.4696) (42.4567, 30.9717) (41.8555, 30.5208) (41.4281, 30.5208) knots 0 0 0 1 2 2 2
  spline S150 degree 2 poles (41.4281, 30.5208) (40.8363, 30.5208) (40.0988, 31.4085) (40.0988, 32.1412) knots 0 0 0 1 2 2 2
  spline S151 degree 2 poles (40.0988, 32.1412) (40.0988, 32.5029) (40.2773, 33.2356) (40.4135, 33.4846) knots 0 0 0 1 2 2 2
  line L86 (40.4135, 33.4846) -> (41.1979, 33.4846)
  line L87 (41.1979, 33.4846) -> (41.1979, 33.447)
  spline S152 degree 2 poles (41.1979, 33.447) (40.9725, 33.1652) (40.7141, 32.4794) (40.7141, 32.1271) knots 0 0 0 1 2 2 2
  spline S153 degree 2 poles (40.7141, 32.1271) (40.7141, 31.7655) (41.0194, 31.2676) (41.3247, 31.2676) knots 0 0 0 1 2 2 2
  spline S154 degree 2 poles (41.3247, 31.2676) (41.6019, 31.2676) (41.8696, 31.5635) (41.9541, 31.8923) knots 0 0 0 1 2 2 2
  spline S155 degree 2 poles (41.9541, 31.8923) (41.9964, 32.052) (42.0809, 32.4559) (42.1326, 32.6767) knots 0 0 0 1 2 2 2
  spline S156 degree 2 poles (42.1326, 32.6767) (42.2547, 33.1558) (42.8137, 33.6443) (43.2974, 33.6443) knots 0 0 0 1 2 2 2
  spline S157 degree 2 poles (43.2974, 33.6443) (43.5793, 33.6443) (44.0771, 33.4235) (44.2603, 33.2074) knots 0 0 0 1 2 2 2
  spline S158 degree 2 poles (44.2603, 33.2074) (44.4529, 32.9773) (44.6548, 32.3902) (44.6548, 31.944) knots 0 0 0 1 2 2 2
  spline S159 degree 2 poles (44.6502, 36.2135) (44.6502, 35.1708) (43.4806, 34.0247) (42.4003, 34.0247) knots 0 0 0 1 2 2 2
  spline S160 degree 2 poles (42.4003, 34.0247) (41.3388, 34.0247) (40.08, 35.1379) (40.08, 36.035) knots 0 0 0 1 2 2 2
  spline S161 degree 2 poles (40.08, 36.035) (40.08, 36.4389) (40.3149, 37.0636) (40.5638, 37.2938) knots 0 0 0 1 2 2 2
  spline S162 degree 2 poles (40.5638, 37.2938) (40.8128, 37.5286) (41.5314, 37.7775) (42.0528, 37.7775) knots 0 0 0 1 2 2 2
  line L88 (42.0528, 37.7775) -> (42.452, 37.7775)
  line L89 (42.452, 37.7775) -> (42.452, 34.7668)
  spline S163 degree 2 poles (42.452, 34.7668) (43.2082, 34.7668) (44.0114, 35.5277) (44.0114, 36.2041) knots 0 0 0 1 2 2 2
  spline S164 degree 2 poles (44.0114, 36.2041) (44.0114, 36.4436) (43.9033, 36.9086) (43.8188, 37.0965) knots 0 0 0 1 2 2 2
  spline S165 degree 2 poles (43.8188, 37.0965) (43.7249, 37.2938) (43.5605, 37.5662) (43.4853, 37.6554) knots 0 0 0 1 2 2 2
  line L90 (43.4853, 37.6554) -> (43.4853, 37.6977)
  line L91 (43.4853, 37.6977) -> (44.2838, 37.6977)
  spline S166 degree 2 poles (44.2838, 37.6977) (44.3355, 37.5709) (44.4858, 37.1857) (44.528, 37.0354) knots 0 0 0 1 2 2 2
  spline S167 degree 2 poles (44.528, 37.0354) (44.5891, 36.8241) (44.6502, 36.4765) (44.6502, 36.2135) knots 0 0 0 1 2 2 2
  spline S168 degree 2 poles (41.8931, 37.0636) (41.5972, 37.0542) (41.165, 36.9321) (41.0194, 36.8147) knots 0 0 0 1 2 2 2
  spline S169 degree 2 poles (41.0194, 36.8147) (40.855, 36.6879) (40.6813, 36.2886) (40.6813, 35.9927) knots 0 0 0 1 2 2 2
  spline S170 degree 2 poles (40.6813, 35.9927) (40.6813, 35.7015) (40.855, 35.2929) (41.0241, 35.1238) knots 0 0 0 1 2 2 2
  spline S171 degree 2 poles (41.0241, 35.1238) (41.1979, 34.9594) (41.6159, 34.7903) (41.8931, 34.7668) knots 0 0 0 1 2 2 2
  line L92 (41.8931, 34.7668) -> (41.8931, 37.0636)
  point P0 (0, 0)
  constraints: 2 other
extrude "Extrusion6" cut sketch "Skizze10" against normal blind 1
